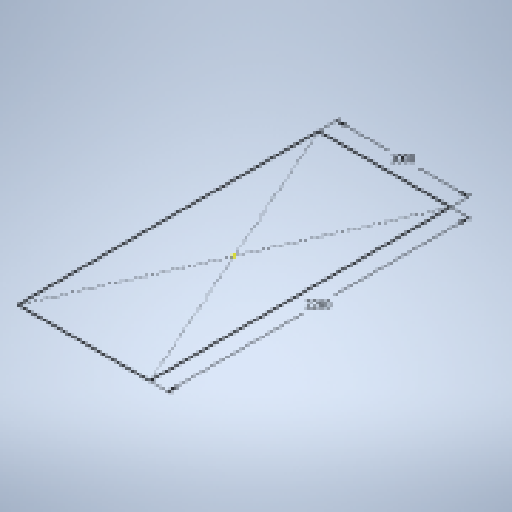
# Autodesk Inventor part: ДМФ 067 крышка
Saved by Autodesk Inventor 2025 (Build 290162010, 162A)
## iProperties
Created: 2024-06-28
Part Number: ДМФ 067 крышка
Material: Generic
Document SubType Name: Sheet Metal
Designer: admin
Density: 1 g/cm^3
Sheet Metal Rule: Default
Appearance: Default
Author: admin
Autodesk Inventor part; units mm, degrees
ref_plane "YZ Plane" through (0, 0, 0) normal (1, 0, 0) x (0, 1, 0)
ref_plane "XZ Plane" through (0, 0, 0) normal (0, 1, 0) x (-1, 0, 0)
ref_plane "XY Plane" through (0, 0, 0) normal (0, 0, 1) x (1, 0, 0)
sketch "Sketch1" plane through (0, 0, 0) normal (0, 0, 1) x (1, 0, 0)
  line L0 (-500, -1140) -> (500, -1140)
  line L1 (500, -1140) -> (500, 1140)
  line L2 (500, 1140) -> (-500, 1140)
  line L3 (-500, 1140) -> (-500, -1140)
  line L4 (-500, -1140) -> (500, 1140) construction
  line L5 (500, -1140) -> (-500, 1140) construction
  point P0 (0, 0)
  dimension "d0" = 1000
  dimension "d1" = 2280
  measures "d0" distance of L2.end L1.end
  measures "d1" distance of L1.end L0.end
extrude "Plate1" add sketch "Sketch1" along normal blind 10
sketch "Sketch2" plane through (0, 0, 10) normal (0, 0, 1) x (1, 0, 0)
  line L0 (500, -1140) -> (-500, -1140) projected
  line L1 (500, 1140) -> (500, -1140) projected
  line L2 (-500, 1140) -> (500, 1140) projected
  line L3 (-500, -1140) -> (-500, 1140) projected
  circle A0 centre (0, -989.5) radius 35
  point P0 (0, 0)
  point P1 (0, -1140)
  dimension "d3" = 70
  dimension "d4" = 150.5
  constraints: 1 centre point, 1 midpoint, 1 vertical alignment
  measures "d3" diameter of A0
  measures "d4" distance from line of L0 A0.centre
extrude "Extrusion1" cut sketch "Sketch2" against normal through all contours A0
pattern_linear "Rectangular Pattern1" count 9 spacing 250 along (0, 1, 0) of "Extrusion1"
equation "\"d2\" = Thickness"
equation "\"BendReliefDepth\" = 0.5 * Thickness"
equation "\"Thickness\" = 10"
body "Solid1"
